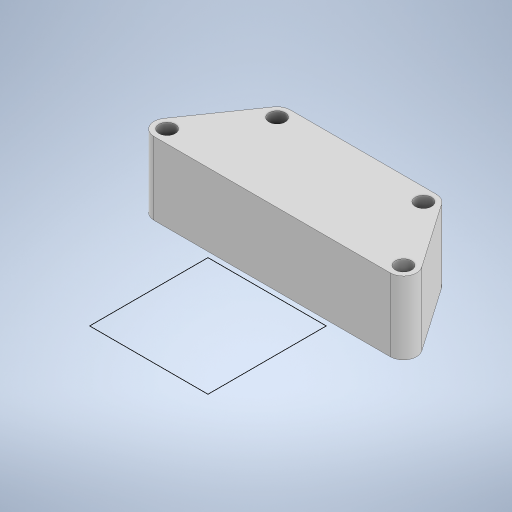
# Autodesk Inventor part: pre camera mount block
Saved by Autodesk Inventor 2023 (Build 270158000, 158)
## iProperties
Created: 2023-01-23
Part Number: pre camera mount block
Material: Generic
Document SubType Name: Modeling
Designer: Steven
Density: 1 g/cm^3
Appearance: Default
Author: Steven
Autodesk Inventor part; units mm, degrees
ref_plane "YZ Plane" through (0, 0, 0) normal (1, 0, 0) x (0, 1, 0)
ref_plane "XZ Plane" through (0, 0, 0) normal (0, 1, 0) x (-1, 0, 0)
ref_plane "XY Plane" through (0, 0, 0) normal (0, 0, 1) x (1, 0, 0)
sketch "Sketch1" plane through (0, 0, 0) normal (0, 1, 0) x (-1, 0, 0)
  circle A0 centre (-72.2448, 0) radius 2.5
  circle A1 centre (-58.4854, -19.8505) radius 2.5
  circle A2 centre (0, 0) radius 2.5
  circle A3 centre (-13.7594, -19.8505) radius 2.5
  line L0 (-54.1974, 5.6029) -> (-18.0474, 5.6029)
  line L1 (-54.1974, 41.7529) -> (-54.1974, 5.6029)
  line L2 (-18.0474, 5.6029) -> (-18.0474, 41.7529)
  line L3 (-18.0474, 41.7529) -> (-54.1974, 41.7529)
  constraints: 8 end point, 4 centre point, 2 horizontal, 2 vertical, 13 other
sketch "Sketch2" plane through (0, 0, 0) normal (0, 1, 0) x (-1, 0, 0)
  circle A0 centre (-72.2448, 0) radius 2.5 projected
  circle A1 centre (-58.4854, -19.8505) radius 2.5 projected
  circle A2 centre (-13.7594, -19.8505) radius 2.5 projected
  circle A3 centre (0, 0) radius 2.5 projected
  circle A4 centre (-72.2448, 0) radius 4
  circle A5 centre (-58.4854, -19.8505) radius 4
  circle A6 centre (-13.7594, -19.8505) radius 4
  circle A7 centre (0, 0) radius 4
  line L0 (-58.4854, -23.8505) -> (-13.7594, -23.8505)
  line L1 (3.2875, -2.2787) -> (-10.4719, -22.1292)
  line L2 (-61.7729, -22.1292) -> (-75.5322, -2.2787)
  line L3 (-72.2448, 4) -> (0, 4)
  dimension "d0" = 8
  dimension "d1" = 8
  dimension "d2" = 8
  dimension "d3" = 8
  constraints: 8 end point, 8 point on circle, 5 tangent, 4 centre point, 4 coincident, 3 horizontal
  measures "d0" diameter of A4
  measures "d1" diameter of A5
  measures "d2" diameter of A6
  measures "d3" diameter of A7
extrude "Extrusion1" add sketch "Sketch2" along normal blind 22.2
body "Solid1"
